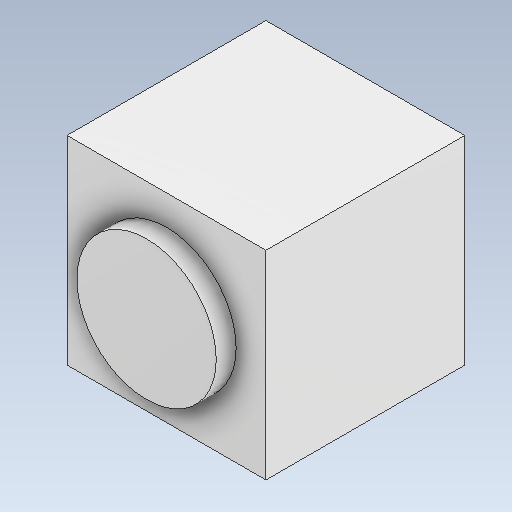
# Autodesk Inventor part: motor
Saved by Autodesk Inventor 2021 (Build 250183000, 183)
## iProperties
Created: 2022-06-27
Part Number: motor
Material: Пластик АБС
Document SubType Name: Modeling
Designer: termi
Density: 1.06 g/cm^3
Appearance: Гладкий - белый
Author: termi
Autodesk Inventor part; units mm, degrees
ref_plane "YZ Plane" through (0, 0, 0) normal (1, 0, 0) x (0, 1, 0)
ref_plane "XZ Plane" through (0, 0, 0) normal (0, 1, 0) x (-1, 0, 0)
ref_plane "XY Plane" through (0, 0, 0) normal (0, 0, 1) x (1, 0, 0)
sketch "Эскиз1" plane through (0, 0, 0) normal (0, 1, 0) x (-1, 0, 0)
  line L0 (-50, 50) -> (50, 50)
  line L1 (50, 50) -> (50, -50)
  line L2 (50, -50) -> (-50, -50)
  line L3 (-50, -50) -> (-50, 50)
  line L4 (-50, 50) -> (50, -50) construction
  line L5 (50, 50) -> (-50, -50) construction
  point P0 (0, 0)
  dimension "d0" = 100
  dimension "d1" = 100
  constraints: 12 end point, 2 midpoint, 2 parallel, 1 horizontal, 1 perpendicular
  measures "d0" distance of L1.end L2.end
  measures "d1" distance of L0.end L1.end
extrude "Выдавливание1" add sketch "Эскиз1" along normal mid plane 100
sketch "Эскиз2" plane through (-50, 50, 50) normal (0, 0, 1) x (1, 0, 0)
  circle A0 centre (50, -50) radius 35
  dimension "d4" = 70
  constraints: 1 centre point, 1 coincident
  measures "d4" diameter of A0
extrude "Выдавливание2" add sketch "Эскиз2" along normal blind 10
